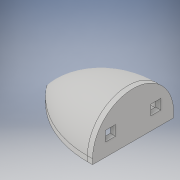
# Autodesk Inventor part: Walllamp
Saved by Autodesk Inventor 2019 (Build 230136000, 136)
## iProperties
Created: 2019-08-18
Part Number: Walllamp
Material: Generic
Document SubType Name: Modeling
Designer: Riley
Density: 1 g/cm^3
Appearance: Default
Author: Riley
Autodesk Inventor part; units mm, degrees
ref_plane "YZ Plane" through (0, 0, 0) normal (1, 0, 0) x (0, 1, 0)
ref_plane "XZ Plane" through (0, 0, 0) normal (0, 1, 0) x (-1, 0, 0)
ref_plane "XY Plane" through (0, 0, 0) normal (0, 0, 1) x (1, 0, 0)
sketch "Sketch3" plane through (0, 0, 0) normal (0, 1, 0) x (-1, 0, 0)
  line L0 (0, 0) -> (0, -6.35)
  line L1 (100.2, -50.1) -> (93.85, -50.1)
  arc A0 (100.2, -50.1) -> (0, 0) centre (-0.4314, -126.1128) ccw
  arc A1 (93.85, -50.1) -> (0, -6.35) centre (1.2123, -126.2853) ccw
  line L2 (93.85, -50.1) -> (0, -50.1) construction
  dimension "d13" = 6.35
  dimension "d15" = 50.1
  dimension "d16" = 6.35
  dimension "d17" = 100.2
  constraints: 6 end point, 4 point on circle, 2 centre point, 2 horizontal, 1 vertical
  measures "d13" distance of L0.start L0.end
  measures "d15" distance of L2.end L0.start
  measures "d16" distance of L1.start L1.end
  measures "d17" distance of L2.end L1.start
revolve "Revolution1" add sketch "Sketch3" angle 180 about axis through (-93.85, 0, -50.1) along (-1, 0, 0)
sketch "Sketch4" plane through (0, 0, -6.35) normal (0, -1, 0) x (1, 0, 0)
  line L0 (0, 6.35) -> (0, 0) projected
  arc A0 (0, 6.35) -> (-100.2, -43.75) centre (0.4314, -119.7628) ccw projected
  arc A1 (-100.2, -43.75) -> (0, -93.85) centre (0.4314, 32.2628) ccw projected
  line L1 (0, -93.85) -> (0, -87.5) projected
  arc A2 (-93.85, -43.75) -> (0, -87.5) centre (-1.2123, 32.4353) ccw projected
  arc A3 (0, 0) -> (-93.85, -43.75) centre (-1.2123, -119.9353) ccw projected
  line L2 (0, 0) -> (0, -87.5) projected
  line L3 (0, -43.75) -> (-100.2, -43.75) construction
  line L4 (-6.35, -18.35) -> (-50.8, -18.35)
  line L5 (-50.8, -69.15) -> (-6.35, -69.15)
  line L6 (-6.35, -69.15) -> (-6.35, -18.35)
  arc A4 (-50.8, -18.35) -> (-50.8, -69.15) centre (-44.9145, -43.75) ccw
  dimension "d21" = 50.8
  dimension "d23" = 25.4
  dimension "d24" = 6.35
  constraints: 8 end point, 2 horizontal, 2 point on circle, 1 centre point, 1 midpoint, 1 parallel
  measures "d21" distance between parallel lines of L5 L4
  measures "d23" distance between parallel lines of L4 L3
  measures "d24" distance between parallel lines of L6 L2
extrude "Extrusion2" add sketch "Sketch4" along normal blind 6.35
sketch "Sketch5" plane through (0, -6.35, 0) normal (1, 0, 0) x (0, 0, -1)
  arc A0 (93.85, 6.35) -> (6.35, 6.35) centre (50.1, 6.35) ccw projected
  line L0 (93.85, 6.35) -> (6.35, 6.35) projected
  line L1 (0, 6.35) -> (0, 0) projected
  line L2 (100.2, 0) -> (0, 0) projected
  line L3 (100.2, 6.35) -> (100.2, 0) projected
  arc A1 (100.2, 6.35) -> (0, 6.35) centre (50.1, 6.35) ccw projected
  line L4 (15.81, 28.8202) -> (28.318, 28.8202)
  line L5 (28.318, 28.8202) -> (28.318, 16.3122)
  line L6 (28.318, 16.3122) -> (15.81, 16.3122)
  line L7 (15.81, 16.3122) -> (15.81, 28.8202)
  line L8 (50.1, 6.35) -> (50.1, 73.5385) construction
  line L9 (84.39, 28.8202) -> (71.882, 28.8202)
  line L10 (71.882, 28.8202) -> (71.882, 16.3122)
  line L11 (71.882, 16.3122) -> (84.39, 16.3122)
  line L12 (84.39, 16.3122) -> (84.39, 28.8202)
  dimension "d28" = 12.508
  dimension "d29" = 12.508
  dimension "d30" = 21.782
  constraints: 18 end point, 4 symmetric about line, 2 parallel, 1 horizontal, 1 perpendicular, 1 vertical
  measures "d28" distance of L5.end L6.end
  measures "d29" distance of L4.end L5.end
  measures "d30" distance between parallel lines of L8 L5
extrude "Extrusion3" add sketch "Sketch5" along normal blind 6.35 contours L0 A0 | A1 L3 L2 L1
equation "\"d16\" = d13"
equation "\"d17\" = 2 * d15"
equation "\"d23\" = 0.5 * d21"
equation "\"d24\" = d13"
equation "\"d26\" = d13"
equation "\"d29\" = d28"
equation "\"d31\" = d13"
body "Solid1"
